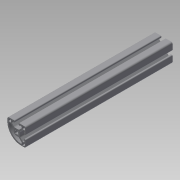
# Autodesk Inventor part: 1517-LS
Saved by Autodesk Inventor 2013 (Build 170138000, 138)
## iProperties
Created: 2014-04-23
Part Number: 1517-LS
Material: Generic
Document SubType Name: Modeling
Density: 1 g/cm^3
Vendor: 80/20 Inc.
Engineer: Ross Bowman
Designer: Ross Bowman
Catalog Web Link: 8020.net
Company: 80/20 Inc.
Author: Ross Bowman
Keywords: 80/20 , 8020 , T-Slot , Extrusion
Material: 6105-T5 Aluminum
Autodesk Inventor part; units mm, degrees
ref_plane "YZ Plane" through (0, 0, 0) normal (1, 0, 0) x (0, 1, 0)
ref_plane "XZ Plane" through (0, 0, 0) normal (0, 1, 0) x (-1, 0, 0)
ref_plane "XY Plane" through (0, 0, 0) normal (0, 0, 1) x (1, 0, 0)
sketch "Sketch1" plane through (0, 0, 0) normal (0, 0, 1) x (1, 0, 0)
  arc A0 (1.8214, -3.4351) -> (3.4385, -1.815) centre (2.63, -2.625) ccw
  line L0 (1.3578, -2.9723) -> (1.8214, -3.4351)
  arc A1 (-1.3522, -2.9748) -> (1.3578, -2.9723) centre (0, 0) ccw
  line L1 (-1.815, -3.4385) -> (-1.3522, -2.9748)
  arc A2 (-3.4351, -1.8214) -> (-1.815, -3.4385) centre (-2.625, -2.63) ccw
  line L2 (-2.9723, -1.3578) -> (-3.4351, -1.8214)
  arc A3 (-2.9748, 1.3522) -> (-2.9723, -1.3578) centre (0, 0) ccw
  line L3 (-3.4385, 1.815) -> (-2.9748, 1.3522)
  arc A4 (-1.8214, 3.4351) -> (-3.4385, 1.815) centre (-2.63, 2.625) ccw
  line L4 (-1.3578, 2.9723) -> (-1.8214, 3.4351)
  arc A5 (1.3522, 2.9748) -> (-1.3578, 2.9723) centre (0, 0) ccw
  line L5 (1.815, 3.4385) -> (1.3522, 2.9748)
  arc A6 (3.4351, 1.8214) -> (1.815, 3.4385) centre (2.625, 2.63) ccw
  line L6 (2.9723, 1.3578) -> (3.4351, 1.8214)
  arc A7 (2.9748, -1.3522) -> (2.9723, 1.3578) centre (0, 0) ccw
  line L7 (3.4385, -1.815) -> (2.9748, -1.3522)
  arc A8 (-15.8829, 8.9846) -> (-8.4146, -8.4146) centre (9.6358, 9.6357) ccw
  arc A9 (-14.6133, 10.287) -> (-15.8829, 8.9846) centre (-14.6133, 9.017) ccw
  line L8 (-12.804, 10.287) -> (-14.6133, 10.287)
  arc A10 (-12.1754, 10.0266) -> (-12.804, 10.287) centre (-12.804, 9.398) ccw
  line L9 (-6.6966, 4.5478) -> (-12.1754, 10.0266)
  arc A11 (-6.3246, 3.6498) -> (-6.6966, 4.5478) centre (-7.5946, 3.6498) ccw
  line L10 (-6.3246, 0) -> (-6.3246, 3.6498)
  arc A12 (-6.3246, 0) -> (0, -6.3246) centre (0, 0) ccw
  line L11 (3.6498, -6.3246) -> (0, -6.3246)
  arc A13 (4.5478, -6.6966) -> (3.6498, -6.3246) centre (3.6498, -7.5946) ccw
  line L12 (10.0266, -12.1754) -> (4.5478, -6.6966)
  arc A14 (10.287, -12.804) -> (10.0266, -12.1754) centre (9.398, -12.804) ccw
  line L13 (10.287, -14.6133) -> (10.287, -12.804)
  arc A15 (8.9846, -15.8829) -> (10.287, -14.6133) centre (9.017, -14.6133) ccw
  arc A16 (-8.4146, -8.4146) -> (8.9846, -15.8829) centre (9.6357, 9.6358) ccw
  arc A17 (14.4522, -17.2466) -> (17.2462, -14.4527) centre (14.4522, -14.4526) ccw
  line L14 (12.2428, -17.2466) -> (14.4522, -17.2466)
  arc A18 (11.8618, -16.8656) -> (12.2428, -17.2466) centre (12.2428, -16.8656) ccw
  line L15 (11.8618, -12.2428) -> (11.8618, -16.8656)
  arc A19 (12.2428, -11.8618) -> (11.8618, -12.2428) centre (12.2428, -12.2428) ccw
  line L16 (16.8653, -11.8618) -> (12.2428, -11.8618)
  arc A20 (17.2463, -12.2428) -> (16.8653, -11.8618) centre (16.8653, -12.2428) ccw
  line L17 (17.2462, -14.4527) -> (17.2463, -12.2428)
  arc A21 (-14.4522, 17.2466) -> (-17.2462, 14.4527) centre (-14.4522, 14.4526) ccw
  line L18 (-12.2428, 17.2466) -> (-14.4522, 17.2466)
  arc A22 (-11.8618, 16.8656) -> (-12.2428, 17.2466) centre (-12.2428, 16.8656) ccw
  line L19 (-11.8618, 12.2428) -> (-11.8618, 16.8656)
  arc A23 (-12.2428, 11.8618) -> (-11.8618, 12.2428) centre (-12.2428, 12.2428) ccw
  line L20 (-16.8653, 11.8618) -> (-12.2428, 11.8618)
  arc A24 (-17.2463, 12.2428) -> (-16.8653, 11.8618) centre (-16.8653, 12.2428) ccw
  line L21 (-17.2462, 14.4527) -> (-17.2463, 12.2428)
  arc A25 (17.2466, 14.4522) -> (14.4527, 17.2462) centre (14.4526, 14.4522) ccw
  line L22 (17.2466, 12.2428) -> (17.2466, 14.4522)
  arc A26 (16.8656, 11.8618) -> (17.2466, 12.2428) centre (16.8656, 12.2428) ccw
  line L23 (12.2428, 11.8618) -> (16.8656, 11.8618)
  arc A27 (11.8618, 12.2428) -> (12.2428, 11.8618) centre (12.2428, 12.2428) ccw
  line L24 (11.8618, 16.8653) -> (11.8618, 12.2428)
  arc A28 (12.2428, 17.2463) -> (11.8618, 16.8653) centre (12.2428, 16.8653) ccw
  line L25 (14.4527, 17.2462) -> (12.2428, 17.2463)
  arc A29 (14.5542, -10.287) -> (15.8242, -9.017) centre (14.5542, -9.017) ccw
  line L26 (14.5542, -10.287) -> (12.9683, -10.287)
  arc A30 (12.0703, -9.915) -> (12.9683, -10.287) centre (12.9683, -9.017) ccw
  line L27 (12.0703, -9.915) -> (8.1222, -5.9669)
  arc A31 (6.731, -2.6083) -> (8.1222, -5.9669) centre (11.4808, -2.6083) ccw
  line L28 (6.731, -2.6083) -> (6.731, 2.6083)
  arc A32 (8.1222, 5.9669) -> (6.731, 2.6083) centre (11.4808, 2.6083) ccw
  line L29 (8.1222, 5.9669) -> (12.0703, 9.915)
  arc A33 (12.9683, 10.287) -> (12.0703, 9.915) centre (12.9683, 9.017) ccw
  line L30 (12.9683, 10.287) -> (14.5542, 10.287)
  arc A34 (15.8242, 9.017) -> (14.5542, 10.287) centre (14.5542, 9.017) ccw
  line L31 (15.8242, 9.017) -> (15.8242, 7.239)
  arc A35 (15.4432, 6.858) -> (15.8242, 7.239) centre (15.4432, 7.239) ccw
  line L32 (15.4432, 6.858) -> (15.367, 6.858)
  arc A36 (15.367, 6.858) -> (14.986, 6.477) centre (15.367, 6.477) ccw
  line L33 (14.986, 6.477) -> (14.986, 5.6388)
  arc A37 (14.986, 5.6388) -> (16.5608, 4.064) centre (16.5608, 5.6388) ccw
  line L34 (16.5608, 4.064) -> (17.4752, 4.064)
  arc A38 (17.4752, 4.064) -> (19.05, 5.6388) centre (17.4752, 5.6388) ccw
  line L35 (19.05, 5.6388) -> (19.05, 15.875)
  arc A39 (19.05, 15.875) -> (15.875, 19.05) centre (15.875, 15.875) ccw
  line L36 (15.875, 19.05) -> (5.6388, 19.05)
  arc A40 (5.6388, 19.05) -> (4.064, 17.4752) centre (5.6388, 17.4752) ccw
  line L37 (4.064, 17.4752) -> (4.064, 16.5608)
  arc A41 (4.064, 16.5608) -> (5.6388, 14.986) centre (5.6388, 16.5608) ccw
  line L38 (5.6388, 14.986) -> (6.477, 14.986)
  arc A42 (6.477, 14.986) -> (6.858, 15.367) centre (6.477, 15.367) ccw
  line L39 (6.858, 15.367) -> (6.858, 15.4432)
  arc A43 (7.239, 15.8242) -> (6.858, 15.4432) centre (7.239, 15.4432) ccw
  line L40 (7.239, 15.8242) -> (9.017, 15.8242)
  arc A44 (10.287, 14.5542) -> (9.017, 15.8242) centre (9.017, 14.5542) ccw
  line L41 (10.287, 14.5542) -> (10.287, 12.9683)
  arc A45 (9.915, 12.0703) -> (10.287, 12.9683) centre (9.017, 12.9683) ccw
  line L42 (9.915, 12.0703) -> (5.9669, 8.1222)
  arc A46 (2.6083, 6.731) -> (5.9669, 8.1222) centre (2.6083, 11.4808) ccw
  line L43 (2.6083, 6.731) -> (-2.6083, 6.731)
  arc A47 (-5.9669, 8.1222) -> (-2.6083, 6.731) centre (-2.6083, 11.4808) ccw
  line L44 (-5.9669, 8.1222) -> (-9.915, 12.0703)
  arc A48 (-10.287, 12.9683) -> (-9.915, 12.0703) centre (-9.017, 12.9683) ccw
  line L45 (-10.287, 12.9683) -> (-10.287, 14.5542)
  arc A49 (-9.017, 15.8242) -> (-10.287, 14.5542) centre (-9.017, 14.5542) ccw
  line L46 (-9.017, 15.8242) -> (-7.239, 15.8242)
  arc A50 (-6.858, 15.4432) -> (-7.239, 15.8242) centre (-7.239, 15.4432) ccw
  line L47 (-6.858, 15.4432) -> (-6.858, 15.367)
  arc A51 (-6.858, 15.367) -> (-6.477, 14.986) centre (-6.477, 15.367) ccw
  line L48 (-6.477, 14.986) -> (-5.6388, 14.986)
  arc A52 (-5.6388, 14.986) -> (-4.064, 16.5608) centre (-5.6388, 16.5608) ccw
  line L49 (-4.064, 16.5608) -> (-4.064, 17.4752)
  arc A53 (-4.064, 17.4752) -> (-5.6388, 19.05) centre (-5.6388, 17.4752) ccw
  line L50 (-5.6388, 19.05) -> (-15.875, 19.05)
  arc A54 (-15.875, 19.05) -> (-19.05, 15.875) centre (-15.875, 15.875) ccw
  line L51 (-19.05, 15.875) -> (-19.05, 9.525)
  arc A55 (-19.05, 9.525) -> (9.525, -19.05) centre (9.525, 9.525) ccw
  line L52 (9.525, -19.05) -> (15.875, -19.05)
  arc A56 (15.875, -19.05) -> (19.05, -15.875) centre (15.875, -15.875) ccw
  line L53 (19.05, -15.875) -> (19.05, -5.6388)
  arc A57 (19.05, -5.6388) -> (17.4752, -4.064) centre (17.4752, -5.6388) ccw
  line L54 (17.4752, -4.064) -> (16.5608, -4.064)
  arc A58 (16.5608, -4.064) -> (14.986, -5.6388) centre (16.5608, -5.6388) ccw
  line L55 (14.986, -5.6388) -> (14.986, -6.477)
  arc A59 (14.986, -6.477) -> (15.367, -6.858) centre (15.367, -6.477) ccw
  line L56 (15.367, -6.858) -> (15.4432, -6.858)
  arc A60 (15.8242, -7.239) -> (15.4432, -6.858) centre (15.4432, -7.239) ccw
  line L57 (15.8242, -7.239) -> (15.8242, -9.017)
  constraints: 122 point on circle, 116 end point, 61 centre point
extrude "Extrusion1" add sketch "Sketch1" against normal blind 304.8
body "Solid1"
